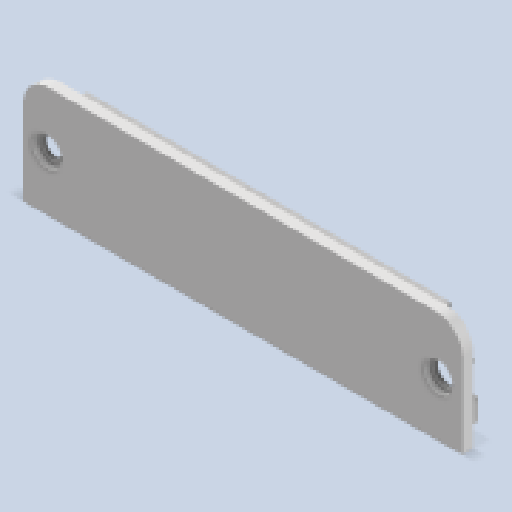
# Autodesk Inventor part: colortop
Saved by Autodesk Inventor 2026.2 (Build 302298000, 298)
## iProperties
Created: 2026-04-10
Part Number: colortop
Material: Generic
Document SubType Name: Modeling
Designer: Fork
Density: 1 g/cm^3
Appearance: Default
Author: Fork
Autodesk Inventor part; units mm, degrees
ref_plane "YZ Plane" through (0, 0, 0) normal (1, 0, 0) x (0, 1, 0)
ref_plane "XZ Plane" through (0, 0, 0) normal (0, 1, 0) x (-1, 0, 0)
ref_plane "XY Plane" through (0, 0, 0) normal (0, 0, 1) x (1, 0, 0)
sketch "Sketch1" plane through (0, 0, 0) normal (0, 0, 1) x (1, 0, 0)
  circle A0 centre (0.25, 36.05) radius 28 projected
  line L0 (-21, -56.05) -> (-21, -1.05) projected
  line L1 (-21, -1.05) -> (21.5, -1.05) projected
  line L2 (21.5, -1.05) -> (21.5, -56.05) projected
  line L3 (21.5, -56.05) -> (-21, -56.05) projected
  arc A1 (-41, -66.05) -> (-36, -71.05) centre (-36, -66.05) ccw projected
  line L4 (-36, -71.05) -> (36, -71.05) projected
  arc A2 (36, -71.05) -> (41, -66.05) centre (36, -66.05) ccw projected
  line L5 (41, -66.05) -> (41, 71.05) projected
  line L6 (41, 71.05) -> (-41, 71.05) projected
  line L7 (-41, 71.05) -> (-41, -66.05) projected
  line L8 (20, 69.05) -> (20, 73.05) projected
  line L9 (20, 69.05) -> (33.3542, 69.05) projected
  arc A3 (33.3542, 69.05) -> (39, 63.4042) centre (36, 66.05) ccw projected
  line L10 (39, 63.4042) -> (39, -63.4042) projected
  arc A4 (39, -63.4042) -> (33.3542, -69.05) centre (36, -66.05) ccw projected
  line L11 (33.3542, -69.05) -> (-33.3542, -69.05) projected
  arc A5 (-33.3542, -69.05) -> (-39, -63.4042) centre (-36, -66.05) ccw projected
  line L12 (-39, -63.4042) -> (-39, 63.4042) projected
  arc A6 (-39, 63.4042) -> (-33.3542, 69.05) centre (-36, 66.05) ccw projected
  line L13 (-33.3542, 69.05) -> (-20, 69.05) projected
  line L14 (-20, 69.05) -> (-20, 73.05) projected
  line L15 (-39, 73.05) -> (-20, 73.05) projected
  line L16 (-39, 79.0505) -> (-39, 73.05) projected
  arc A7 (-34, 89.95) -> (-39, 84.95) centre (-34, 84.95) ccw projected
  line L17 (34, 89.95) -> (-34, 89.95) projected
  arc A8 (39, 84.95) -> (34, 89.95) centre (34, 84.95) ccw projected
  line L18 (39, 73.05) -> (39, 79.0505) projected
  line L19 (20, 73.05) -> (39, 73.05) projected
  line L20 (41, -66.05) -> (41, 86.95) projected
  arc A9 (41, 86.95) -> (36, 91.95) centre (36, 86.95) ccw projected
  line L21 (-36, 91.95) -> (36, 91.95) projected
  arc A10 (-36, 91.95) -> (-41, 86.95) centre (-36, 86.95) ccw projected
  line L22 (-41, -66.05) -> (-41, 86.95) projected
  arc A11 (-41, -66.05) -> (-36, -71.05) centre (-36, -66.05) ccw projected
  line L23 (-36, -71.05) -> (36, -71.05) projected
  arc A12 (36, -71.05) -> (41, -66.05) centre (36, -66.05) ccw projected
  circle A13 centre (-36, -66.05) radius 2.1 projected
  line L24 (38.6458, 69.05) -> (39, 69.05) projected
  line L25 (39, 69.05) -> (39, 68.6958) projected
  arc A14 (39, 68.6958) -> (38.6458, 69.05) centre (36, 66.05) ccw projected
  circle A15 centre (36, 66.05) radius 2.1 projected
  line L26 (39, -68.6958) -> (39, -69.05) projected
  line L27 (39, -69.05) -> (38.6458, -69.05) projected
  arc A16 (38.6458, -69.05) -> (39, -68.6958) centre (36, -66.05) ccw projected
  circle A17 centre (36, -66.05) radius 2.1 projected
  arc A18 (-39, -68.6958) -> (-38.6458, -69.05) centre (-36, -66.05) ccw projected
  line L28 (-38.6458, -69.05) -> (-39, -69.05) projected
  line L29 (-39, -69.05) -> (-39, -68.6958) projected
  circle A19 centre (-36, 66.05) radius 2.1 projected
  arc A20 (-38.6458, 69.05) -> (-39, 68.6958) centre (-36, 66.05) ccw projected
  line L30 (-39, 68.6958) -> (-39, 69.05) projected
  line L31 (-39, 69.05) -> (-38.6458, 69.05) projected
  line L32 (41, 71.25) -> (-41, 71.25)
  circle A21 centre (-36.5, 81.5) radius 2.1 projected
  circle A22 centre (36.5, 81.5) radius 2.1 projected
  arc A23 (-39, 79.0505) -> (-39, 83.9495) centre (-36.5, 81.5) ccw projected
  line L33 (-39, 84.95) -> (-39, 83.9495) projected
  line L34 (39, 83.9495) -> (39, 84.95) projected
  arc A24 (39, 83.9495) -> (39, 79.0505) centre (36.5, 81.5) ccw projected
  point P0 (0, 0)
  dimension "d0" = 0.2
  constraints: 2 end point, 2 point on line, 1 perpendicular
  measures "d0" distance between parallel lines of L6 L32
extrude "Extrusion1" add sketch "Sketch1" along normal blind 2 contours L22 A10 L21 A9 L20 L32 L8 L19 L18 A24 L34 A8 L17 A7 L33 A23 L16 L15 L14 | L14 L15 L16 A23 L33 A7 L17 A8 L34 A24 L18 L19 L8 L32 | A21 | A22
sketch "Sketch2" plane through (0, 0, 0) normal (0, 0, -1) x (-1, 0, 0)
  arc A0 (-34, 89.95) -> (-39, 79.0505) centre (-34, 84.95) ccw projected
  line L0 (-34, 89.95) -> (34, 89.95) projected
  arc A1 (39, 79.0505) -> (34, 89.95) centre (34, 84.95) ccw projected
  line L1 (39, 79.0505) -> (39, 73.05) projected
  line L2 (-39, 73.05) -> (-39, 79.0505) projected
  line L3 (38.9, 73.05) -> (38.9, 84.95)
  arc A2 (38.9, 84.95) -> (34, 89.85) centre (34, 84.95) ccw
  line L4 (34, 89.85) -> (-34, 89.85)
  arc A3 (-34, 89.85) -> (-38.9, 84.95) centre (-34, 84.95) ccw
  line L5 (-38.9, 84.95) -> (-38.9, 73.05)
  line L6 (-37.9, 73.05) -> (-37.9, 84.95)
  arc A4 (-34, 88.85) -> (-37.9, 84.95) centre (-34, 84.95) ccw
  line L7 (-34, 88.85) -> (34, 88.85)
  arc A5 (37.9, 84.95) -> (34, 88.85) centre (34, 84.95) ccw
  line L8 (37.9, 84.95) -> (37.9, 73.05)
  line L9 (-38.9, 73.05) -> (-37.9, 73.05)
  line L10 (37.9, 73.05) -> (38.9, 73.05)
  line L11 (41, 71.25) -> (-41, 71.25) projected
  arc A6 (-34, 89.95) -> (-39, 84.95) centre (-34, 84.95) ccw projected
  line L12 (-34, 89.95) -> (34, 89.95) projected
  circle A7 centre (-36.5, 81.5) radius 2.1 projected
  arc A8 (-39, 79.0505) -> (-39, 83.9495) centre (-36.5, 81.5) ccw projected
  circle A9 centre (36.5, 81.5) radius 2.1 projected
  arc A10 (39, 83.9495) -> (39, 79.0505) centre (36.5, 81.5) ccw projected
  arc A11 (-36, 91.95) -> (-41, 86.95) centre (-36, 86.95) ccw projected
  line L13 (-41, 71.25) -> (-41, 86.95) projected
  line L14 (-34, 88.85) -> (-34, 89.95)
  line L15 (-38.9, 77.05) -> (38.9, 77.05)
  line L16 (34, 89.95) -> (34, 88.85)
  point P0 (0, 0)
  point P1 (-38.4, 73.05)
  point P2 (38.4, 73.05)
  point P3 (-37.9, 83.0652)
  point P4 (-38.3525, 82.4891)
  point P5 (-37.9, 81.8211)
  point P6 (38.3525, 82.4891)
  point P7 (37.9, 83.0652)
  point P8 (37.9, 81.8211)
  point P9 (-37.9, 77.05)
  point P10 (37.9, 77.05)
  point P11 (34, 89.85)
  dimension "d3" = 0.1
  dimension "d4" = 1
  dimension "d5" = 16.8
  dimension "d6" = 16.8
  dimension "d15" = 2.1
  dimension "d16" = 4
  constraints: 22 end point, 8 point on circle, 4 centre point, 2 midpoint, 2 perpendicular, 2 point on line, 1 horizontal, 1 parallel, 1 vertical, 10 other
  measures "d3" distance between parallel lines of L0 L4
  measures "d4" radial gap between concentric circles of A3 A4
  measures "d5" vertical distance of L4.start L8.end
  measures "d6" vertical distance of L4.end point (-38.4, 73.05)
  measures "d15" distance between parallel lines of L13 L5
  measures "d16" distance from line of point (38.4, 73.05) L15
extrude "Extrusion2" add sketch "Sketch2" along normal blind 3 contours L4 L16 L7 L14 | L3 L10 L8 L15 | L15 L6 L9 L5
sketch "Sketch3" plane through (0, 0, 2) normal (0, 0, 1) x (1, 0, 0)
  circle A0 centre (36.5, 81.5) radius 2.1 projected
  circle A1 centre (-36.5, 81.5) radius 2.1 projected
  point P0 (0, 0)
extrude "Extrusion3" cut sketch "Sketch3" against normal blind 3
sketch "Sketch4" plane through (0, 0, 2) normal (0, 0, 1) x (1, 0, 0)
  circle A0 centre (36.5, 81.5) radius 2.1 projected
  circle A1 centre (36.5, 81.5) radius 2.75
  circle A2 centre (-36.5, 81.5) radius 2.1 projected
  circle A3 centre (-36.5, 81.5) radius 2.75
  point P0 (0, 0)
  point P1 (-37.9, 79.9348)
  point P2 (-37.9, 83.0652)
  dimension "d11" = 5.5
  dimension "d12" = 5.5
  constraints: 2 centre point, 2 coincident
  measures "d11" diameter of A1
  measures "d12" diameter of A3
extrude "Extrusion4" cut sketch "Sketch4" against normal blind 1 contours A0 | A1 | A2 | A3
body "Solid1"
